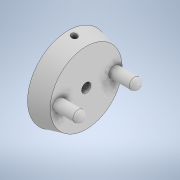
# Autodesk Inventor part: volante final
Saved by Autodesk Inventor 2022.1 (Build 261234020, 234B)
## iProperties
Created: 2023-08-18
Part Number: volante final
Material: Generic
Document SubType Name: Modeling
Designer: SENAI
Density: 1 g/cm^3
Appearance: Default
Author: SENAI
Autodesk Inventor part; units mm, degrees
ref_plane "YZ Plane" through (0, 0, 0) normal (1, 0, 0) x (0, 1, 0)
sketch "Sketch1" plane through (0, 0, 0) normal (0, 0, 1) x (1, 0, 0)
  line L0 (0, 0) -> (0, 22)
  line L1 (0, 22) -> (25, 22)
  line L2 (25, 22) -> (25, 71)
  line L3 (25, 71) -> (6, 71)
  line L4 (6, 71) -> (6, 75)
  line L5 (6, 75) -> (0, 75)
  line L6 (37, 0) -> (37, 73.5)
  line L7 (0, 75) -> (0, 83)
  line L8 (0, 83) -> (37, 73.5)
  line L9 (0, 0) -> (37, 0)
  dimension "d0" = 22
  dimension "d1" = 25
  dimension "d2" = 49
  dimension "d3" = 19
  dimension "d4" = 4
  dimension "d6" = 37
  dimension "d7" = 73.5
  dimension "d8" = 8
  dimension "d9" = 104.4
  constraints: 20 end point, 4 perpendicular, 2 horizontal, 2 vertical, 1 parallel
  measures "d0" distance of L0.start L0.end
  measures "d1" distance of L0.end L1.end
  measures "d2" distance of L1.end L2.end
  measures "d3" distance of L2.end L3.end
  measures "d4" distance of L3.end L4.end
  measures "d6" distance of L0.start L6.start
  measures "d7" distance of L6.start L6.end
  measures "d8" distance of L5.end L7.end
  measures "d9" angle of L8 L6
revolve "Revolution1" add sketch "Sketch1" angle 360 about axis through (0, 0, 0) along (1, 0, 0)
sketch "Sketch2" plane through (0, 0, 0) normal (-1, 0, 0) x (0, 0, 1)
  circle A0 centre (0, 0) radius 9.5
  dimension "d11" = 19
  constraints: 1 centre point, 1 coincident
  measures "d11" diameter of A0
extrude "Extrusion1" cut sketch "Sketch2" against normal blind 37
sketch "Sketch3" plane through (37, 0, 0) normal (1, 0, 0) x (0, 0, -1)
  point P0 (0, 0)
sketch "Sketch4" plane through (25, 0, 0) normal (-1, 0, 0) x (0, 0, 1)
  point P0 (0, 0)
ref_plane "Work Plane1" through (12.5, 22, 0) normal (0, 1, 0) x (-1, 0, 0)
sketch "Sketch5" plane through (12.5, 22, 0) normal (0, 1, 0) x (-1, 0, 0)
  point P0 (12.5, 0)
  point P1 (0, 0)
  point P2 (0, 0)
  point P3 (0, 0)
  constraints: 2 coincident
sketch "Sketch6" plane through (37, 0, 0) normal (1, 0, 0) x (0, 0, -1)
  circle A0 centre (-57.5, 0) radius 11.25
  circle A1 centre (57.5, 0) radius 11.25
  point P0 (0, 0)
  dimension "d15" = 22.5
  dimension "d16" = 22.5
  constraints: 2 centre point
  measures "d15" diameter of A0
  measures "d16" diameter of A1
extrude "Extrusion2" add sketch "Sketch6" along normal blind 52.5
fillet "Fillet1" radius 11 2 edges at (89.5, 0, 68.75) (89.5, 0, -46.25)
hole "Hole1" at (12.5, 22, 0) direction (0, -1, 0) diameter 9 depth 45 tip angle 118
sketch "Sketch7" plane through (12.5, 22, 0) normal (0, 1, 0) x (-1, 0, 0)
  point P0 (12.5, 0)
  point P1 (0, 0)
  point P2 (0, 0)
  constraints: 1 coincident
hole "Hole2" at (12.5, 22, 0) direction (0, 1, 0) diameter 12 end through all
ref_plane "Work Plane2" through (12.5, -22, 0) normal (0, 1, 0) x (-1, 0, 0)
sketch "Sketch8" plane through (12.5, -22, 0) normal (0, 1, 0) x (-1, 0, 0)
  point P0 (12.5, 0)
  point P1 (0, 0)
  point P2 (0, 0)
  constraints: 1 coincident
hole "Hole3" at (12.5, -22, 0) direction (0, -1, 0) diameter 12 end through all
body "Solid1"
